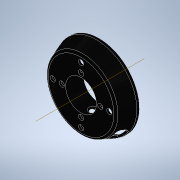
# Autodesk Inventor part: Base
Saved by Autodesk Inventor 2022 (Build 260153000, 153)
## iProperties
Created: 2022-09-16
Part Number: Base
Material: Stainless Steel
Document SubType Name: Modeling
Designer: Nathan Cai
Density: 8 g/cm^3
Appearance: Anodized - Black
Author: Nathan Cai
Autodesk Inventor part; units mm, degrees
ref_plane "XY Plane" through (0, 0, 0) normal (0, 0, 1) x (1, 0, 0)
sketch "Sketch1" plane through (0, 0, 0) normal (1, 0, 0) x (0, 1, 0)
  line L0 (0, 0) -> (31.5, 0)
  line L1 (31.5, 0) -> (31.5, -14)
  line L2 (31.5, -14) -> (0, -14)
  line L3 (0, -14) -> (0, 0) construction
  line L4 (27, 0) -> (31.5, -12)
  line L5 (0, 0) -> (12, 0)
  line L6 (12, 0) -> (12, -14)
  line L7 (12, -14) -> (0, -14)
  line L8 (0, -14) -> (0, 0) construction
  dimension "d0" = 31.5
  dimension "d1" = 14
  dimension "d2" = 2
  dimension "d3" = 27
  dimension "d4" = 12
  constraints: 18 end point, 4 parallel, 3 point on line, 2 horizontal, 2 perpendicular
  measures "d0" distance of L1.end L2.end
  measures "d1" distance of L0.end L1.end
  measures "d2" distance from line of L2 L4.end
  measures "d3" distance from line of L3 L4.start
  measures "d4" distance of L6.end L7.end
revolve "Revolution1" add sketch "Sketch1" angle 360 about axis through (0, 0, -14) along (0, 0, 1) contours L0 L4 L1 L2 L6
fillet "Fillet1" radius 2 1 edges at (0, -27, 0)
shell "Shell1" thickness 1.5875 removed faces 1 at (2.5128, 24.6949, -14)
sketch "Sketch2" plane through (0, 0, 0) normal (0, 0, 1) x (1, 0, 0)
  circle A0 centre (0, 0) radius 15 construction
  circle A1 centre (0, 0) radius 22 construction
  line L0 (0, 0) -> (0, 22) construction
  circle A2 centre (0, 15) radius 2
  circle A3 centre (0, 22) radius 2
  circle A4 centre (-22, 0) radius 2
  circle A5 centre (-15, 0) radius 2
  circle A6 centre (0, -22) radius 2
  circle A7 centre (0, -15) radius 2
  circle A8 centre (22, 0) radius 2
  circle A9 centre (15, 0) radius 2
  dimension "d7" = 30
  dimension "d8" = 44
  dimension "d9" = 4
  dimension "d10" = 4
  dimension "d13" = 360
  constraints: 8 centre point, 3 coincident, 2 end point, 2 vertical alignment, 1 point on line, 1 vertical, 21 other
  measures "d9" diameter of A2
  measures "d10" diameter of A3
extrude "Extrusion1" cut sketch "Sketch2" against normal blind 25.4
ref_plane "Work Plane1" through (0, 0, 0) normal (-0.7071, 0.7071, 0) x (0, 0, 1)
sketch "Sketch3" plane through (0, 0, 0) normal (-0.7071, 0.7071, 0) x (0, 0, 1)
  line L0 (-14, 8.6088) -> (-14, -8.6088) projected
  line L1 (-14, 0) -> (0, 0) construction
  line L2 (-7, -5) -> (-7, 5) construction
  line L3 (-14, 8.6088) -> (-1.5875, 8.6088) projected
  line L4 (-3, -5) -> (-3, 5)
  line L5 (-11, 5) -> (-11, -5)
  arc A0 (-11, -5) -> (-3, -5) centre (-7, -5) ccw
  arc A1 (-3, 5) -> (-11, 5) centre (-7, 5) ccw
  line L6 (-7, 0) -> (3, 0) construction
  point P0 (-5.2748, 8.6088)
  point P1 (-8.7252, 8.6088)
  dimension "d18" = 5
  dimension "d19" = 90
  dimension "d20" = 8
  constraints: 12 end point, 4 point on circle, 4 tangent, 3 midpoint, 2 centre point, 2 horizontal, 2 perpendicular, 1 parallel
  measures "d18" distance of L6.start L2.end
  measures "d19" angle of L6 L2
  measures "d20" diameter of A1
extrude "Extrusion2" cut sketch "Sketch3" against normal blind 50.8 contours L3 A1 L4 A0 L5
body "Solid1"
